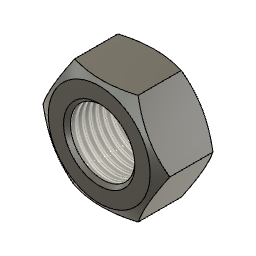
gaika (Autodesk Fusion 360 design; units mm, degrees)
Autodesk Fusion 360 part; units mm, degrees
sketch "Sketch1" plane through (0, 0, 0) normal (0, 0, 1) x (1, 0, 0) in component "Гайка Гост 10605-94"
  line L0 (23.094, 40) -> (46.188, 0)
  line L1 (-23.094, 40) -> (23.094, 40)
  line L2 (-46.188, 0) -> (-23.094, 40)
  line L3 (-23.094, -40) -> (-46.188, 0)
  line L4 (23.094, -40) -> (-23.094, -40)
  line L5 (46.188, 0) -> (23.094, -40)
extrude "Extrude1" add sketch "Sketch1" along normal blind 42 in component "Гайка Гост 10605-94"
sketch "Sketch2" plane through (0, 0, 0) normal (0, 1, 0) x (1, 0, 0) in component "Гайка Гост 10605-94"
  line L0 (37.1, 0) -> (92.376, 0)
  line L1 (92.376, 0) -> (92.376, -31.9136)
  line L2 (92.376, -31.9136) -> (37.1, 0)
revolve "Revolve1" cut sketch "Sketch2" angle 360 about axis through (0, 0, 1.75) along (0, 0, 1) in component "Гайка Гост 10605-94"
ref_plane "WorkPlane1" through (0, 0, 21) normal (0, 0, 1) x (1, 0, 0) in component "Гайка Гост 10605-94"
mirror "Mirror1" about plane through (0, 0, 21) normal (0, 0, 1) of "Revolve1" in component "Гайка Гост 10605-94"
sketch "Sketch3" plane through (0, 0, 0) normal (0, 0, 1) x (1, 0, 0) in component "Гайка Гост 10605-94"
  circle A0 centre (0, 0) radius 26
extrude "Extrude2" cut sketch "Sketch3" along normal blind 42 in component "Гайка Гост 10605-94"
thread "Thread1" "ISO Metric profile 52.0 M52x5 6H" major diameter 52.5183 minor diameter 46.9423 pitch 5 angle 60 resizes the face on face at (25.9677, -1.296, 28) in component "Гайка Гост 10605-94"
chamfer "Chamfer1" distance 2.529 angle 45 1 edges at (-21.8828, 8.4875, 42) in component "Гайка Гост 10605-94"
mirror "Mirror2" about plane through (0, 0, 21) normal (0, 0, 1) of 1 faces at (25.1259, -1.254, 41.157) in component "Гайка Гост 10605-94"
component "Гайка Гост 10605-94" placed x (1, 0, 0) y (0, 1, 0) z (0, 0, 1) at (0, 0, 0)
equation "distanceOne = 42.00 mm"
equation "taperAngle1 = 0.0 deg"
equation "angle = 360.0 deg"
equation "offset = 21.00 mm"
equation "StitchTolerance = 0.01 mm"
equation "distance = 2.529 mm"
